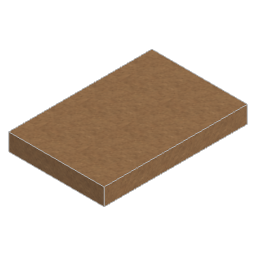
_Europalette Standard.2801aa45-2bc8-4bd9-9d11-928ec4eb7075 (Autodesk Fusion 360 design; units mm, degrees)
Autodesk Fusion 360 part; units mm, degrees
sketch "Sketch1" plane through (0, 0, 0) normal (0, 0, 1) x (1, 0, 0)
  line L0 (-36.1073, 33.6313) -> (763.8927, 33.6313)
  line L1 (763.8927, 33.6313) -> (763.8927, -1166.3687)
  line L2 (763.8927, -1166.3687) -> (-36.1073, -1166.3687)
  line L3 (-36.1073, -1166.3687) -> (-36.1073, 33.6313)
  dimension "d1" = 800
  dimension "d2" = 1200
  constraint horizontal L0
  constraint vertical L1
  constraint horizontal L2
  constraint vertical L3
  measures "d1" distance of L0.start L0.end
  measures "d2" distance of L0.start L2.end
extrude "Extrude1" add sketch "Sketch1" along normal blind 144
